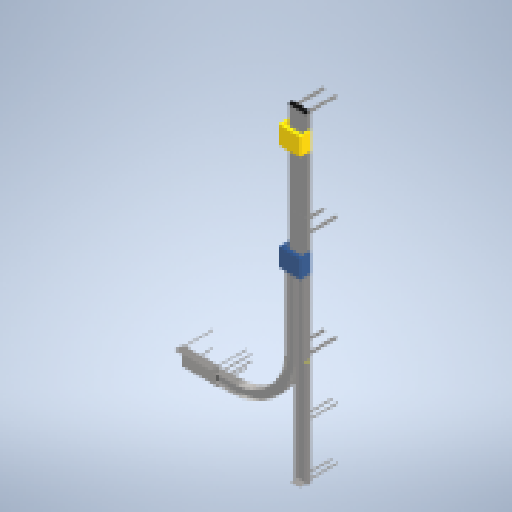
# Autodesk Inventor part: ConveyorS&F
Saved by Autodesk Inventor 2025.1 (Build 291241000, 241)
## iProperties
Created: 2025-02-25
Part Number: ConveyorS&F
Material: Generic
Document SubType Name: Modeling
Designer: yovan
Density: 1 g/cm^3
Appearance: Default
Author: yovan
Autodesk Inventor part; units mm, degrees
ref_plane "YZ Plane" through (0, 0, 0) normal (1, 0, 0) x (0, 1, 0)
ref_plane "XZ Plane" through (0, 0, 0) normal (0, 1, 0) x (-1, 0, 0)
ref_plane "XY Plane" through (0, 0, 0) normal (0, 0, 1) x (1, 0, 0)
sketch "Sketch1" plane through (0, 0, 0) normal (1, 0, 0) x (0, 1, 0)
  line L0 (60, 0) -> (5940, 0)
  line L1 (5940, 120) -> (60, 120)
  arc A0 (60, 120) -> (60, 0) centre (60, 60) ccw
  arc A1 (5940, 0) -> (5940, 120) centre (5940, 60) ccw
  line L2 (60, 0) -> (110, 0)
  line L3 (110, 0) -> (110, -780)
  line L4 (110, -780) -> (60, -780)
  line L5 (60, -780) -> (60, 0)
  line L6 (5940, 0) -> (5890, 0)
  line L7 (5890, 0) -> (5890, -780)
  line L8 (5890, -780) -> (5940, -780)
  line L9 (5940, -780) -> (5940, 0)
  line L10 (3025, -780) -> (2975, -780)
  line L11 (2975, -780) -> (2975, 0)
  line L12 (2975, 0) -> (3025, 0)
  line L13 (3025, 0) -> (3025, -780)
  point P0 (0, 0)
  dimension "d2" = 50
  dimension "d3" = 780
  dimension "d4" = 50
  dimension "d5" = 780
  dimension "d8" = 50
  constraints: 28 end point, 7 parallel, 4 horizontal, 4 point on circle, 3 perpendicular, 2 centre point, 1 point on line
  measures "d2" distance of L3.end L4.end
  measures "d3" distance of L2.end L3.end
  measures "d4" distance of L8.end L7.end
  measures "d5" distance of L7.end L6.end
  measures "d8" distance of L11.end L12.end
extrude "Extrusion1" add sketch "Sketch1" along normal blind 50 contours A0 L1 A1 L0
extrude "Extrusion2" add sketch "Sketch1" against normal blind 400 contours A0 L1 A1 L0
extrude "Extrusion3" add sketch "Sketch1" against normal blind 50 contours L0 L3 L4 L5 | L0 L13 L10 L11 | L9 L8 L7 L0
sketch "Sketch2" plane through (-400, 0, 0) normal (-1, 0, 0) x (0, 0, 1)
  line L0 (-780, 110) -> (-780, 60) projected
  line L1 (-780, 110) -> (0, 110)
  line L2 (0, 110) -> (0, 60)
  line L3 (0, 60) -> (-780, 60)
  line L4 (-780, 60) -> (-780, 110)
  line L5 (0, 3025) -> (-780, 3025) projected
  line L6 (-780, 2975) -> (0, 2975) projected
  line L7 (-780, 3025) -> (0, 3025)
  line L8 (0, 3025) -> (0, 2975)
  line L9 (0, 2975) -> (-780, 2975)
  line L10 (-780, 2975) -> (-780, 3025)
  line L11 (0, 5890) -> (-780, 5890) projected
  line L12 (0, 5940) -> (-780, 5940) projected
  line L13 (-780, 5890) -> (0, 5890)
  line L14 (0, 5890) -> (0, 5940)
  line L15 (0, 5940) -> (-780, 5940)
  line L16 (-780, 5940) -> (-780, 5890)
  arc A0 (120, 5940) -> (0, 5940) centre (60, 5940) ccw projected
  circle A1 centre (60, 5940) radius 60
  arc A2 (0, 60) -> (120, 60) centre (60, 60) ccw projected
  circle A3 centre (60, 60) radius 60
  line L17 (120, 60) -> (120, 5940)
  line L18 (0, 5940) -> (0, 60) projected
  line L19 (0, 5940) -> (0, 60)
  point P0 (0, 0)
  constraints: 28 end point, 7 equal length, 4 vertical, 3 horizontal, 3 perpendicular, 2 coincident, 2 horizontal alignment, 4 other
extrude "Extrusion4" add sketch "Sketch2" against normal blind 50 contours L1 L2 L3 L0 | L6 L10 L5 L8 | L11 L16 L12 L14
extrude "Extrusion5" add sketch "Sketch2" along normal blind 50 contours L18 L8 L14 A1 L17 A3 L2 | A3 A2 | A1 A0
sketch "Sketch3" plane through (50, 60, 120) normal (0, 0, 1) x (1, 0, 0)
  line L0 (-100, 0) -> (-400, 0) projected
  line L1 (-250, 0) -> (1750, 0) construction
  line L2 (-500, -60) -> (0, -60) projected
  line L3 (-245, 2000) -> (-255, 2000)
  line L4 (-255, 2000) -> (-255, -60)
  line L5 (-255, -60) -> (-245, -60)
  line L6 (-245, -60) -> (-245, 2000)
  point P0 (-50, -60)
  dimension "d21" = 10
  constraints: 10 end point, 2 horizontal, 2 parallel, 1 midpoint, 1 perpendicular, 1 point on line
  measures "d21" distance of L5.end L4.end
extrude "Extrusion6" add sketch "Sketch3" along normal blind 100
extrude "Extrusion7" cut sketch "Sketch3" along normal blind 5
sketch "Sketch4" plane through (50, 60, 120) normal (0, 0, 1) x (1, 0, 0)
  line L0 (0, -60) -> (0, 0) projected
  line L1 (0, 0) -> (-250, 0)
  line L2 (-250, 0) -> (-250, -3060)
  line L3 (-250, -3060) -> (0, -3060)
  line L4 (0, -3060) -> (0, 0)
  line L5 (-250, -3060) -> (-250, 0)
  arc A0 (-2030, -1530) -> (-500, 0) centre (-2030, 0) ccw
  arc A1 (-2030, -1780) -> (-250, 0) centre (-2030, 0) ccw
  line L6 (-450, 0) -> (-500, 0) projected
  line L7 (-500, 0) -> (-250, 0)
  line L8 (-100, 0) -> (-400, 0) projected
  line L9 (-2530, -1530) -> (-2030, -1530)
  line L10 (-2030, -1780) -> (-2530, -1780)
  line L11 (-2530, -1780) -> (-2530, -1530)
  line L12 (-2030, 0) -> (-250, 0) construction
  circle A2 centre (-40, -2980) radius 20
  circle A3 centre (-210, -2980) radius 20
  circle A4 centre (-2450, -1740) radius 20
  circle A5 centre (-2450, -1570) radius 20
  circle A6 centre (-1129.485, -1286.0687) radius 20
  circle A7 centre (-1031.9774, -1425.324) radius 20.0003
  circle A8 centre (-40, -1530) radius 20
  circle A9 centre (-210, -1530) radius 20
  line L13 (-2030, -1540) -> (-2520, -1540)
  line L14 (-2520, -1540) -> (-2520, -1770)
  line L15 (-2520, -1770) -> (-2030, -1770)
  arc A10 (-2030, -1540) -> (-490.0325, -10) centre (-2030, 0) ccw
  line L16 (-490.0325, -10) -> (-250, -10)
  arc A11 (-2030, -1770) -> (-260, 0) centre (-2030, 0) ccw
  line L17 (-10, -10) -> (-240, -10)
  line L18 (-240, -10) -> (-240, -3050)
  line L19 (-240, -3050) -> (-10, -3050)
  line L20 (-10, -3050) -> (-10, -10)
  line L21 (-10, -10) -> (-10, 2000)
  line L22 (-10, 2000) -> (0, 2000)
  line L23 (0, 2000) -> (0, 0)
  line L24 (-490.0325, -10) -> (-500.0325, -10)
  line L25 (-500.0325, -10) -> (-500.0325, 2000)
  line L26 (-500.0325, 2000) -> (-490.0325, 2000)
  line L27 (-490.0325, 2000) -> (-490.0325, -10)
  dimension "d30" = 250
  dimension "d31" = 3060
  dimension "d73" = 10
  dimension "d74" = 10
  dimension "d75" = 10
  dimension "d76" = 10
  dimension "d77" = 10
  dimension "d78" = 2010
  constraints: 50 end point, 12 centre point, 8 parallel, 8 point on circle, 4 horizontal, 4 perpendicular, 2 collinear, 1 midpoint, 1 vertical, 6 other
  measures "d30" distance of L3.end L2.end
  measures "d31" distance of L2.end L1.end
  measures "d73" distance between parallel lines of L9 L13
  measures "d74" radial gap between concentric circles of A0 A10
  measures "d75" radial gap between concentric circles of A1 A11
  measures "d76" distance between parallel lines of L4 L20
  measures "d77" distance of L25.end L26.end
  measures "d78" distance of L24.end L25.end
extrude "Extrusion8" add sketch "Sketch4" against normal blind 120 contours L4 L3 L2 L1 L0 | A1 L16 A11 L7 | A1 L10 L11 L9 A0 L24 A10 L13 L14 L15 A11 L16 | A11 L16 L27 L6 L7 | A11 L15 L14 L13 A10 L16 | L24 A0 L6 L27 | A2 | A3 | A4 | A5 | A6 | A7 | A8 | A9 | L20 L19 L18 L17
fillet "Fillet1" radius 60 4 edges at (-75, -3000, 120) (-75, -3000, 0) (-2480, -1595, 120) (-2480, -1595, 0)
extrude "Extrusion9" add sketch "Sketch4" against normal blind 900 contours A2 | A3 | A4 | A5 | A6 | A7 | A8 | A9
sketch "Sketch5" plane through (-1980, -1720, 0) normal (0, -1, 0) x (1, 0, 0)
  line L0 (-510, 60) -> (-1510, 60)
  line L1 (-510, 60) -> (490, 60) construction
  line L2 (-1510, 60) -> (-510, 60)
  line L3 (-510, 60) -> (-510, 30)
  line L4 (-510, 30) -> (-1510, 30)
  line L5 (-1510, 30) -> (-1510, 60)
  point P0 (1980, 0)
  dimension "d57" = 1000
  dimension "d58" = 180
  dimension "d59" = 30
  constraints: 12 end point, 3 horizontal, 2 parallel, 1 collinear, 1 perpendicular
  measures "d57" distance of L0.start L0.end
  measures "d58" angle of L0 L1
  measures "d59" distance of L2.end L3.end
extrude "Extrusion10" add sketch "Sketch5" against normal blind 300
extrude "Extrusion11" add sketch "Sketch5" along normal blind 200
sketch "Sketch6" plane through (-450, 5940, 120) normal (0, 0, 1) x (1, 0, 0)
  line L0 (250, -8940) -> (250, -8880) projected
  line L1 (250, -8880) -> (500, -8880)
  line L2 (500, -8880) -> (500, -8870)
  line L3 (500, -8870) -> (250, -8870)
  line L4 (250, -8870) -> (250, -8880)
  point P0 (450, -5940)
  dimension "d64" = 250
  dimension "d65" = 10
  constraints: 8 end point, 2 parallel, 1 horizontal, 1 perpendicular
  measures "d64" distance of L3.end L2.end
  measures "d65" distance of L2.end L1.end
extrude "Extrusion12" add sketch "Sketch6" along normal blind 200
extrude "Extrusion13" cut sketch "Sketch6" along normal blind 5
sketch "Sketch7" plane through (-3490, -1420, 60) normal (0, 0, 1) x (1, 0, 0)
  line L0 (0, 0) -> (1000, 0) projected
  line L1 (1000, 0) -> (1000, -500) projected
  line L2 (0, 0) -> (1000, 0)
  line L3 (1000, 0) -> (1000, -10)
  line L4 (1000, -10) -> (0, -10)
  line L5 (0, -10) -> (0, 0)
  point P0 (3490, 1420)
  dimension "d70" = 10
  constraints: 8 end point, 2 parallel, 1 horizontal, 1 perpendicular, 1 point on line
  measures "d70" distance of L2.end L3.end
extrude "Extrusion14" add sketch "Sketch7" along normal blind 200
sketch "Sketch8" plane through (-450, 5940, 120) normal (0, 0, 1) x (1, 0, 0)
  point P0 (450, -5940)
sketch "Sketch9" plane through (-450, 5940, 120) normal (0, 0, 1) x (1, 0, 0)
  line L0 (-43.4774, -3880) -> (546.7965, -3880)
  line L1 (0, 0) -> (0, -5880) projected
  line L2 (0, -3880) -> (10, -3880)
  line L3 (10, -3880) -> (10, -5940)
  line L4 (10, -5940) -> (0, -5940)
  line L5 (0, -5940) -> (0, -3880)
  line L6 (500, 0) -> (500, -8880) projected
  line L7 (500, -3880) -> (490, -3880)
  line L8 (490, -3880) -> (490, -5940)
  line L9 (490, -5940) -> (500, -5940)
  line L10 (500, -5940) -> (500, -3880)
  arc A0 (-1530, -7410) -> (0, -5880) centre (-1530, -5880) ccw projected
  arc A1 (-1530, -7410) -> (0, -5880) centre (-1530, -5880) ccw
  line L11 (245, -5940) -> (255, -5940) projected
  line L12 (245, -5940) -> (248.9885, -5940)
  line L13 (245, -5940) -> (248.9885, -5940)
  arc A2 (-1470, -7420) -> (11.1684, -5880) centre (-1530, -5880) ccw
  line L14 (11.1684, -5880) -> (11.1684, 0)
  line L15 (-1530, -7410) -> (-1970, -7410)
  line L16 (-1970, -7410) -> (-1970, -7420)
  line L17 (-1970, -7420) -> (-1470, -7420)
  line L18 (-1970, -7660) -> (-1970, -7410) projected
  line L19 (-1530, -7660) -> (-1970, -7660)
  line L20 (-1970, -7660) -> (-1970, -7650)
  line L21 (-1970, -7650) -> (-1590, -7655)
  arc A3 (-1590, -7655) -> (245, -5940) centre (-1530, -5880) ccw
  arc A4 (-1530, -7660) -> (248.9885, -5940) centre (-1530, -5880) ccw
  arc A5 (11.1684, -4989.3822) -> (0, -4970.3297) centre (-1530, -5880) ccw
  line L22 (490, -5940) -> (500, -5940)
  line L23 (500, -5940) -> (500, -8869.955)
  line L24 (500, -8869.955) -> (490, -8869.955)
  line L25 (490, -8869.955) -> (490, -5940)
  line L26 (255, -5940) -> (250, -5940)
  line L27 (250, -5940) -> (250, -8869.955)
  line L28 (250, -8869.955) -> (255, -8869.955)
  line L29 (255, -8869.955) -> (255, -5940)
  dimension "d79" = 10
  dimension "d80" = 10
  dimension "d82" = 11.1684
  dimension "d83" = 10
  dimension "d84" = 10
  constraints: 52 end point, 11 point on line, 10 point on circle, 8 horizontal, 8 parallel, 6 perpendicular, 5 centre point, 1 coincident, 1 other
  measures "d79" distance of L3.end L4.end
  measures "d80" distance of L9.end L8.end
  measures "d82" radial gap between concentric circles of A0 A2
  measures "d83" distance of L15.end L16.end
  measures "d84" distance of L18.start L20.end
extrude "Extrusion15" add sketch "Sketch9" along normal blind 100 contours L0 L3 A5 L1 | A5 L3 L4 L5 L1 | L5 L4 A2 L17 L16 L15 A0 | L0 L6 L9 L8 | L11 A4 L19 L18 L21 A3 | L11 L29 L28 L27
extrude "Extrusion16" add sketch "Sketch9" along normal blind 30 contours L9 L6 L24 L25
sketch "Sketch10" plane through (-2490, -1420, 30) normal (0, 0, -1) x (-1, 0, 0)
  circle A0 centre (970, -470) radius 15
  circle A1 centre (970, -30) radius 15
  circle A2 centre (30, -470) radius 15
  circle A3 centre (30, -30) radius 15
  point P0 (-2490, 1420)
  point P1 (1000, -500)
  point P2 (0, -500)
  constraints: 4 centre point
extrude "Extrusion17" add sketch "Sketch10" along normal blind 810
sketch "Sketch12" plane through (-450, 5940, 120) normal (0, 0, 1) x (1, 0, 0)
  point P0 (450, -5940)
ref_plane "Work Plane1" through (-200, 5560, 320) normal (0, -1, 0) x (1, 0, 0)
sketch "Sketch13" plane through (-200, 5560, 320) normal (0, -1, 0) x (1, 0, 0)
  line L0 (300, -260) -> (-300, -260)
  line L1 (-300, -260) -> (-300, 40)
  line L2 (-300, 40) -> (300, 40)
  line L3 (300, 40) -> (300, -260)
  line L4 (-250, -60) -> (-250, -210)
  line L5 (-250, -210) -> (250, -210)
  line L6 (250, -210) -> (250, -60)
  line L7 (-250, -60) -> (250, -60)
  point P0 (200, -320)
  dimension "d98" = 600
  dimension "d99" = 300
  constraints: 16 end point, 3 parallel, 2 perpendicular, 1 horizontal
  measures "d98" distance of L1.end L2.end
  measures "d99" distance of L0.end L1.end
extrude "Extrusion18" add sketch "Sketch13" along normal blind 500
ref_plane "Work Plane2" through (-200, 2560, 320) normal (0, -1, 0) x (1, 0, 0)
sketch "Sketch14" plane through (-200, 2560, 320) normal (0, -1, 0) x (1, 0, 0)
  line L0 (300, -260) -> (300, 40) projected
  line L1 (300, 40) -> (-300, 40) projected
  line L2 (300, -260) -> (-300, -260)
  line L3 (-300, -260) -> (-300, 40)
  line L4 (-300, 40) -> (300, 40)
  line L5 (300, 40) -> (300, -260)
  line L6 (250, -260) -> (250, -60)
  line L7 (-250, -60) -> (250, -60)
  line L8 (-250, -60) -> (-250, -210)
  line L9 (-250, -210) -> (250, -210)
  line L10 (250, -210) -> (250, -60)
  point P0 (200, -320)
  constraints: 18 end point, 3 parallel, 2 perpendicular, 1 horizontal, 1 point on line
extrude "Extrusion19" add sketch "Sketch14" along normal blind 450
extrude "Extrusion20" add sketch "Sketch14" against normal blind 50
sketch "Sketch15" plane through (-450, 5940, 120) normal (0, 0, 1) x (1, 0, 0)
  line L0 (0, -3880) -> (0, -3830) projected
  line L1 (500, -3830) -> (500, -3880) projected
  line L2 (0, -3855) -> (500, -3855)
  line L3 (500, -3855) -> (500, -3860)
  line L4 (500, -3860) -> (0, -3860)
  line L5 (0, -3860) -> (0, -3855)
  point P0 (450, -5940)
  dimension "d111" = 5
  constraints: 8 end point, 2 parallel, 1 horizontal, 1 midpoint, 1 perpendicular, 1 point on line
  measures "d111" distance of L2.end L3.end
extrude "Extrusion21" cut sketch "Sketch15" against normal blind 120
extrude "Extrusion22" cut sketch "Sketch3" against normal blind 120
sketch "Sketch16" plane through (-200, -2940, 120) normal (0, 0, 1) x (1, 0, 0)
  line L0 (5, 5000) -> (-5, 5000) projected
  line L1 (-5, 5000) -> (5, 5000)
  line L2 (5, 5000) -> (5, 5022.9803)
  line L3 (5, 5022.9803) -> (-5, 5022.9803)
  line L4 (-5, 5022.9803) -> (-5, 5000)
  point P0 (200, 2940)
  dimension "d116" = 10
  constraints: 8 end point, 2 parallel, 1 horizontal, 1 perpendicular
  measures "d116" distance of L3.end L2.end
extrude "Extrusion23" cut sketch "Sketch16" against normal blind 120
sketch "Sketch17" plane through (-450, 5940, 120) normal (0, 0, 1) x (1, 0, 0)
  line L0 (0, -2500) -> (500, -2500)
  line L1 (500, -2500) -> (500, -2505)
  line L2 (500, -2505) -> (0, -2505)
  line L3 (0, -2505) -> (0, -2500)
  point P0 (450, -5940)
  dimension "d119" = 500
  dimension "d120" = 5
  constraints: 8 end point, 2 parallel, 1 horizontal, 1 perpendicular
  measures "d119" distance of L1.end L2.end
  measures "d120" distance of L0.end L1.end
extrude "Extrusion24" cut sketch "Sketch17" against normal blind 120
body "Solid1"
